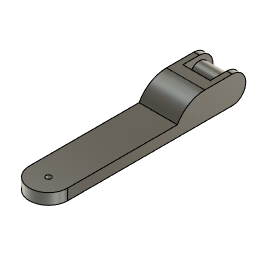
IndexFingerLeftGear v1 (Autodesk Fusion 360 design; units mm, degrees)
Autodesk Fusion 360 part; units mm, degrees
sketch "Sketch1" plane through (0, 0, 0) normal (0, 0, 1) x (1, 0, 0)
  circle A0 centre (0, 0) radius 7
  line L0 (-7, 0) -> (-7, 50.081)
  line L1 (-7, 50.081) -> (7, 50.081)
  line L2 (7, 50.081) -> (7, 0)
  dimension "d1" = 14
  dimension "d2" = 50.081
  dimension "d3" = 14
  dimension "d4" = 50.081
  constraint coincident A0.centre origin
  constraint coincident A0 L0.start
  constraint vertical L0
  constraint perpendicular L0 L1
  constraint coincident A0 L2.end
  constraint tangent A0 L2
  measures "d1" diameter of A0
  measures "d2" distance of L0.start L0.end
  measures "d3" distance of L0.end L1.end
  measures "d4" vertical distance of L1.end L2.end
extrude "Extrude1" add sketch "Sketch1" along normal blind 4
hole "Hole1" at (0, 0, 4) direction (0, 0, -1) diameter 2 end through all
sketch "Sketch4" plane through (0, 0, 4) normal (0, 0, 1) x (-1, 0, 0)
  circle A0 centre (0, 0) radius 1
  arc A1 (7, 0) -> (-7, 0) centre (0, 0) ccw
  line L0 (-7, 0) -> (-7, -50.081)
  line L1 (-7, -50.081) -> (7, -50.081)
  line L2 (7, -50.081) -> (7, 0)
  line L3 (-7, -50.081) -> (-7, -40.081)
  line L4 (7, -40.081) -> (7, -50.081)
  line L5 (-7, -40.081) -> (7, -40.081)
  dimension "d17" = 10
  constraint coincident L0.end L1.start
  constraint coincident L0 L3.end
  constraint perpendicular L1 L3
  constraint coincident L2 L4.start
  constraint coincident L1.end L2.start
  constraint perpendicular L1 L4
  constraint perpendicular L4 L5
  measures "d17" distance of L4.start L1.end
extrude "Extrude4" add sketch "Sketch4" along normal blind 6 contours L0 L1 L2 L3 L4 L5
fillet "Fillet1" radius 11.5 1 edges at (0, 40.081, 10)
sketch "Sketch5" plane through (-7, 0, 0) normal (-1, 0, 0) x (0, -1, 0)
  arc A0 (-40.081, 4) -> (-50.081, 10) centre (-50.1807, -1.4996) ccw
  line L0 (-50.081, 10) -> (-50.081, 0)
  line L1 (-50.081, 0) -> (0, 0)
  line L2 (0, 0) -> (0, 4)
  line L3 (0, 4) -> (-40.081, 4)
  line L4 (-50.081, 10) -> (-60.081, 10)
  line L5 (-60.081, 10) -> (-60.081, 0)
  line L6 (-60.081, 0) -> (-50.081, 0)
  dimension "d22" = 10
  constraint coincident A0.end L0.start
  constraint perpendicular L0 L4
  constraint perpendicular L4 L5
  constraint coincident L0.end L1.start
  constraint perpendicular L0 L6
  measures "d22" distance of A0.end L4.end
extrude "Extrude5" add sketch "Sketch5" against normal blind 2 contours L0 L4 L5 L6
sketch "Sketch6" plane through (7, 0, 0) normal (1, 0, 0) x (0, 1, 0)
  arc A0 (50.081, 10) -> (40.081, 4) centre (50.1807, -1.4996) ccw
  line L0 (40.081, 4) -> (0, 4)
  line L1 (0, 4) -> (0, 0)
  line L2 (0, 0) -> (50.081, 0)
  line L3 (50.081, 0) -> (50.081, 10)
  line L4 (50.081, 10) -> (60.081, 10)
  line L5 (60.081, 10) -> (60.081, 0)
  line L6 (60.081, 0) -> (50.081, 0)
  dimension "d25" = 10
  constraint coincident A0.start L3.end
  constraint perpendicular L3 L4
  constraint perpendicular L4 L5
  constraint coincident L2.end L3.start
  constraint perpendicular L3 L6
  measures "d25" distance of A0.start L4.end
extrude "Extrude6" add sketch "Sketch6" against normal blind 2 contours L3 L4 L5 L6
sketch "Sketch7" plane through (7, 0, 0) normal (1, 0, 0) x (0, 1, 0)
  arc A0 (50.081, 10) -> (40.081, 4) centre (50.1807, -1.4996) ccw
  line L0 (40.081, 4) -> (0, 4)
  line L1 (0, 4) -> (0, 0)
  line L2 (0, 0) -> (60.081, 0)
  line L3 (60.081, 0) -> (60.081, 10)
  line L4 (60.081, 10) -> (50.081, 10)
  circle A1 centre (60.081, 5) radius 5
  dimension "d28" = 10
  constraint midpoint L3 A1.centre
  measures "d28" diameter of A1
extrude "Extrude7" add sketch "Sketch7" against normal blind 2 contours L3 A1 picked at (62.1497, 5.5371)
sketch "Sketch8" plane through (-7, 0, 0) normal (-1, 0, 0) x (0, -1, 0)
  arc A0 (-40.081, 4) -> (-50.081, 10) centre (-50.1807, -1.4996) ccw
  line L0 (-50.081, 10) -> (-60.081, 10)
  line L1 (-60.081, 10) -> (-60.081, 0)
  line L2 (-60.081, 0) -> (0, 0)
  line L3 (0, 0) -> (0, 4)
  line L4 (0, 4) -> (-40.081, 4)
  circle A1 centre (-60.081, 5) radius 5
  dimension "d31" = 10
  constraint midpoint L1 A1.centre
  measures "d31" diameter of A1
extrude "Extrude8" add sketch "Sketch8" against normal blind 2 contours L1 A1 picked at (-61.9543, 4.6477)
sketch "Sketch9" plane through (0, 50.081, 0) normal (0, 1, 0) x (-1, 0, 0)
  line L0 (-5, 10) -> (-5, 0)
  line L1 (-5, 0) -> (5, 0)
  line L2 (5, 0) -> (5, 10)
  line L3 (5, 10) -> (-5, 10)
extrude "Extrude9" add 1 faces at (1.6667, 50.081, 6.6664) along direction (0, 1, 0) blind 4
sketch "Sketch10" plane through (5, 0, 0) normal (-1, 0, 0) x (0, -1, 0)
  line L0 (-54.081, 0) -> (-54.081, 10)
  line L1 (-54.081, 10) -> (-60.081, 10)
  arc A0 (-60.081, 10) -> (-60.081, 0) centre (-60.081, 5) ccw
  line L2 (-60.081, 0) -> (-54.081, 0)
  circle A1 centre (-60.081, 5) radius 3.25
  dimension "d36" = 6.5
  constraint concentric A0 A1
  measures "d36" diameter of A1
extrude "Extrude10" add sketch "Sketch10" along normal through all of body 1 contours A1
